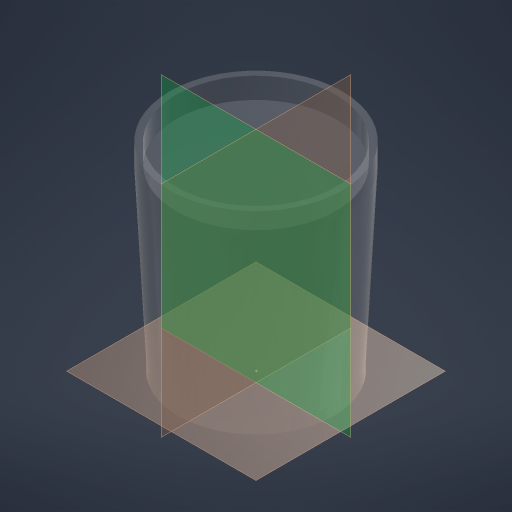
# Autodesk Inventor part: Glas - Reservoir
Saved by Autodesk Inventor 2024 (Build 280153000, 153)
## iProperties
Manager: Louis Van Roosmaelen
Company: DCS - DIGITAL COMBAT SIMULATOR
Created: 2023-11-03
Part Number: Glas - Reservoir
Material: S235
Catalog Web Link: http://emmausbovenbouw.op-weg.be/
Vendor: Emmaüsinstituut Bovenbouw Aalter
Document SubType Name: Modeling
Designer: Louis
Engineer: Declercq St.
Manufacturer: Standard
Standards Organization: Custom
Density: 7.86 g/cm^3
Appearance: Polycarbonate - Clear
IDENT.NR.: AJ2022
TEAM: 30
Title: F18C Home Cockpit
Author: Louis
Keywords: Ø
Autodesk Inventor part; units mm, degrees
sketch "Sketch1" plane through (0, 0, 0) normal (0, 0, 1) x (1, 0, 0)
  line L0 (0, 2.8582) -> (0, -2.8582) construction
  line L1 (-5.7775, 0) -> (5.7775, 0) construction
  circle A0 centre (0, 0) radius 37
  dimension "d0" = 74
  constraints: 4 end point, 2 coincident, 2 midpoint, 1 centre point, 1 horizontal, 1 vertical
  measures "d0" diameter of A0
extrude "Extrusion1" add sketch "Sketch1" along normal blind 5
sketch "Sketch2" plane through (0, 0, 0) normal (0, 1, 0) x (-1, 0, 0)
  line L0 (37, 5) -> (37, 0) projected
  line L1 (37, 0) -> (-37, 0) projected
  line L2 (-37, 0) -> (-37, 5) projected
  line L3 (-37, 5) -> (37, 5) projected
  line L4 (0, 0) -> (0, 85)
  line L5 (0, 85) -> (41, 85)
  line L6 (41, 85) -> (41, 95)
  line L7 (38, 85) -> (38, 95)
  line L8 (38, 95) -> (41, 95)
  line L9 (37, 5) -> (41, 85)
  line L10 (38, 85) -> (34, 5)
  point P0 (0, 5)
  dimension "d4" = 85
  dimension "d5" = 41
  dimension "d6" = 38
  dimension "d7" = 10
  dimension "d8" = 10
  constraints: 14 end point, 3 vertical, 2 point on line, 1 horizontal, 1 parallel
  measures "d4" distance of L4.start L4.end
  measures "d5" distance of L4.end L5.end
  measures "d6" distance from line of L4 L7.start
  measures "d7" distance of L5.end L6.end
  measures "d8" distance of L7.start L7.end
revolve "Revolution1" add sketch "Sketch2" angle 360 about axis through (0, 0, 0) along (0, 0, 1) contours L3 L10 L5 L9 | L3 L4 L5 L10 | L5 L7 L8 L6
body "Solid1"
